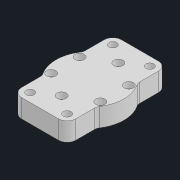
# Autodesk Inventor part: Part1
Saved by Autodesk Inventor 2022 (Build 260153000, 153)
## iProperties
Created: 2021-08-26
Part Number: Part1
Material: 一般
Document SubType Name: Modeling
Designer: Yuta Kage
Density: 1 g/cm^3
Appearance: 既定
Author: Yuta Kage
Autodesk Inventor part; units mm, degrees
ref_plane "YZ Plane" through (0, 0, 0) normal (1, 0, 0) x (0, 1, 0)
ref_plane "XZ Plane" through (0, 0, 0) normal (0, 1, 0) x (-1, 0, 0)
ref_plane "XY Plane" through (0, 0, 0) normal (0, 0, 1) x (1, 0, 0)
sketch "スケッチ1" plane through (0, 0, 0) normal (0, 1, 0) x (-1, 0, 0)
  line L0 (27.5, 27.5) -> (-27.5, 27.5)
  line L1 (-27.5, 27.5) -> (-27.5, -27.5)
  line L2 (-27.5, -27.5) -> (27.5, -27.5)
  line L3 (27.5, -27.5) -> (27.5, 27.5)
  line L4 (27.5, 27.5) -> (-27.5, -27.5) construction
  line L5 (-27.5, 27.5) -> (27.5, -27.5) construction
  line L6 (15, 33.5) -> (-15, 33.5) construction
  line L7 (-15, 33.5) -> (-15, -33.5) construction
  line L8 (-15, -33.5) -> (15, -33.5) construction
  line L9 (15, -33.5) -> (15, 33.5) construction
  line L10 (15, 33.5) -> (-15, -33.5) construction
  line L11 (-15, 33.5) -> (15, -33.5) construction
  circle A0 centre (-15, 33.5) radius 5 construction
  circle A1 centre (0, 0) radius 27.5
  line L12 (22, -40.5) -> (-22, -40.5)
  line L13 (-22, -40.5) -> (-22, 40.5)
  line L14 (-22, 40.5) -> (22, 40.5)
  line L15 (22, 40.5) -> (22, -40.5)
  line L16 (22, -40.5) -> (-22, 40.5) construction
  line L17 (-22, -40.5) -> (22, 40.5) construction
  point P0 (-22, -16.5)
  point P1 (22, -16.5)
  point P2 (22, 16.5)
  point P3 (-22, 16.5)
  dimension "d44" = 55
  dimension "d45" = 10
  dimension "d46" = 6
  dimension "d53" = 55
  dimension "d54" = 30
  dimension "d55" = 7
  dimension "d56" = 7
  constraints: 36 end point, 6 midpoint, 6 parallel, 3 horizontal, 3 perpendicular, 2 centre point, 2 coincident, 1 tangent
  measures "d44" distance between parallel lines of L0 L2
  measures "d45" diameter of A0
  measures "d46" distance from line of L0 A0.centre
  measures "d53" diameter of A1
  measures "d54" distance of L6.start L6.end
  measures "d55" distance from line of A0.centre L13
  measures "d56" distance from line of L14 A0.centre
extrude "押し出し1" add sketch "スケッチ1" along normal mid plane 15 contours L15 A1 L0 | L0 L13 L14 L15 | A1 L15 | A1 L13 L0 | A1 L15 L13 | L15 L2 A1 | L13 A1 | L15 L12 L13 L2 | L2 L13 A1
sketch "スケッチ2" plane through (-1, 7.5, 27) normal (0, -1, 0) x (1, 0, 0)
  line L0 (-14, -60.5) -> (16, -60.5)
  line L1 (16, -60.5) -> (16, 6.5)
  line L2 (16, 6.5) -> (-14, 6.5)
  line L3 (-14, 6.5) -> (-14, -60.5)
  line L4 (-14, -60.5) -> (16, 6.5) construction
  line L5 (16, -60.5) -> (-14, 6.5) construction
  line L6 (-21, 13.5) -> (23, 13.5) projected
  point P0 (1, -27)
  dimension "d52" = 30
  dimension "d58" = 7
  constraints: 12 end point, 2 midpoint, 2 parallel, 1 horizontal, 1 perpendicular
  measures "d52" distance of L0.start L0.end
  measures "d58" distance between parallel lines of L6 L2
hole "穴1" at (-15, 7.5, 33.5) at (15, 7.5, 33.5) at (15, 7.5, -33.5) at (-15, 7.5, -33.5) direction (0, -1, 0) diameter 6.4 end through all clearance for "Flat Head Machine Screw" size "M6" standard "Ansi Metric M Profile"
sketch "スケッチ5" plane through (-26, 7.5, 26) normal (0, 1, 0) x (1, 0, 0)
  circle A0 centre (26, 26) radius 23
  point P0 (26, 26)
  point P1 (26, 49)
  point P2 (26, 26)
  point P3 (6.0814, 37.5)
  point P4 (26, 26)
  point P5 (6.0814, 14.5)
  point P6 (26, 26)
  point P7 (26, 3)
  point P8 (26, 26)
  point P9 (45.9186, 14.5)
  point P10 (26, 26)
  point P11 (45.9186, 37.5)
  dimension "d31" = 46
  dimension "d34" = 360
  constraints: 8 coincident, 2 vertical alignment, 19 other
hole "穴4" at (19.9186, 7.5, -11.5) at (19.9186, 7.5, 11.5) at (0, 7.5, 23) at (-19.9186, 7.5, 11.5) at (-19.9186, 7.5, -11.5) at (0, 7.5, -23) direction (0, -1, 0) diameter 4.3 end through all counterbore diameter 7.5 counterbore depth 5 clearance for "Socket Head Cap Screw" size "M4" standard "Ansi Metric M Profile"
fillet "フィレット2" radius 7 4 edges at (-22, 0, 40.5) (22, 0, 40.5) (22, 0, -40.5) (-22, 0, -40.5)
fillet "フィレット3" radius 5 4 edges at (-22, 0, -16.5) (-22, 0, 16.5) (22, 0, -16.5) (22, 0, 16.5)
